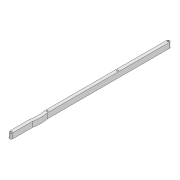
# Autodesk Inventor part: Part_3
Saved by Autodesk Inventor 2022 (Build 260153000, 153)
## iProperties
Created: 2022-05-03
Part Number: Part_3
Material: Generic
Document SubType Name: Modeling
Designer: dell
Density: 1 g/cm^3
Appearance: Default
Author: dell
Autodesk Inventor part; units mm, degrees
ref_plane "YZ Plane" through (0, 0, 0) normal (1, 0, 0) x (0, 1, 0)
ref_plane "XZ Plane" through (0, 0, 0) normal (0, 1, 0) x (-1, 0, 0)
ref_plane "XY Plane" through (0, 0, 0) normal (0, 0, 1) x (1, 0, 0)
sketch "Sketch1" plane through (0, 0, 0) normal (0, 1, 0) x (-1, 0, 0)
  line L0 (0, 0) -> (0, -296.686) construction
  line L1 (-3, 0) -> (-3, -296.686)
  line L2 (3, -296.686) -> (3, 0)
  arc A0 (3, 0) -> (-3, 0) centre (0, 0) ccw
  arc A1 (-3, -296.686) -> (3, -296.686) centre (0, -296.686) ccw
  circle A2 centre (0, 0) radius 1.5
  circle A3 centre (0, -296.686) radius 1.5
  circle A4 centre (0, -200.914) radius 1.5
  circle A5 centre (0, -68.172) radius 1.5
  arc A6 (3, -38.172) -> (3, -65.172) centre (61.4615, -51.672) ccw
  arc A7 (-3, -38.172) -> (-3, -65.172) centre (55.4615, -51.672) ccw
  point P0 (0, -148.343)
  dimension "d0" = 6
  dimension "d1" = 296.686
  dimension "d2" = 3
  dimension "d3" = 3
  dimension "d6" = 3
  dimension "d7" = 200.914
  dimension "d8" = 3
  dimension "d9" = 68.172
  dimension "d10" = 60
  dimension "d11" = 3
  dimension "d12" = 30
  dimension "d13" = 60
  constraints: 8 centre point, 8 end point, 8 point on circle, 6 point on line, 4 tangent, 2 coincident, 2 horizontal alignment, 1 midpoint, 1 parallel, 1 vertical
  measures "d0" diameter of A1
  measures "d1" distance of L0.end L0.start
  measures "d2" diameter of A2
  measures "d3" diameter of A3
  measures "d6" diameter of A4
  measures "d7" distance of L0.start A4.centre
  measures "d8" diameter of A5
  measures "d9" distance of L0.start A5.centre
  measures "d10" radius of A6
  measures "d11" horizontal distance of A5.centre A6.end
  measures "d12" vertical distance of A5.centre A6.start
  measures "d13" radius of A7
extrude "Extrusion1" add sketch "Sketch1" along normal blind 10 contours A0 L2 A6 A1 L1 | L1 A7
body "Solid1"
